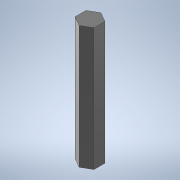
# Autodesk Inventor part: drive hex shaft
Saved by Autodesk Inventor 2022 (Build 260153000, 153)
## iProperties
Created: 2023-01-11
Part Number: drive hex shaft
Material: Generic
Document SubType Name: Modeling
Designer: s135320
Density: 1 g/cm^3
Appearance: Default
Author: s135320
Autodesk Inventor part; units mm, degrees
ref_plane "YZ Plane" through (0, 0, 0) normal (1, 0, 0) x (0, 1, 0)
ref_plane "XZ Plane" through (0, 0, 0) normal (0, 1, 0) x (-1, 0, 0)
ref_plane "XY Plane" through (0, 0, 0) normal (0, 0, 1) x (1, 0, 0)
sketch "Sketch1" plane through (0, 0, 0) normal (0, 1, 0) x (-1, 0, 0)
  line L0 (0, -7.3406) -> (-6.3571, -3.6703)
  line L1 (-6.3571, -3.6703) -> (-6.3571, 3.6703)
  line L2 (-6.3571, 3.6703) -> (0, 7.3406)
  line L3 (0, 7.3406) -> (6.3571, 3.6703)
  line L4 (6.3571, 3.6703) -> (6.3571, -3.6703)
  line L5 (6.3571, -3.6703) -> (0, -7.3406)
  point P0 (0, 0)
  point P1 (0, 0)
  dimension "d0" = 7.3406
  constraints: 12 end point, 1 coincident, 13 other
  measures "d0" distance of L3.end L4.end
extrude "Extrusion1" add sketch "Sketch1" along normal blind 82.55
body "Solid1"
